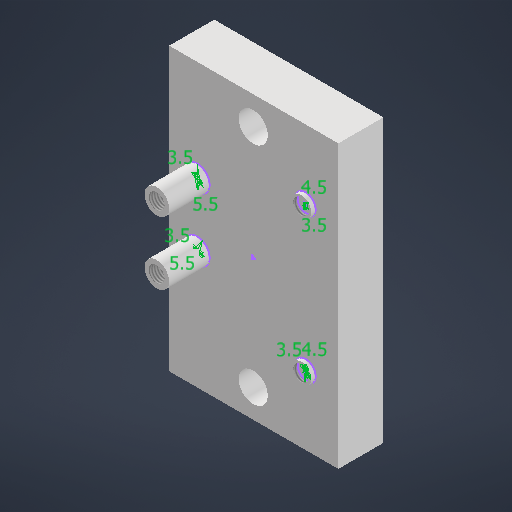
# Autodesk Inventor part: phm_top
Saved by Autodesk Inventor 2027 (Build 310192060, 192F)
## iProperties
Created: 2026-06-05
Part Number: phm_top
Material: Generic
Document SubType Name: Modeling
Designer: jacob
Density: 1 g/cm^3
Appearance: Default
Author: jacob
Autodesk Inventor part; units mm, degrees
ref_plane "YZ Plane" through (0, 0, 0) normal (1, 0, 0) x (0, 1, 0)
ref_plane "XZ Plane" through (0, 0, 0) normal (0, 1, 0) x (-1, 0, 0)
ref_plane "XY Plane" through (0, 0, 0) normal (0, 0, 1) x (1, 0, 0)
sketch "Sketch2" plane through (0, 0, 0) normal (0, 0, 1) x (1, 0, 0)
  line L0 (18.75, -31.25) -> (18.75, 31.25)
  line L1 (18.75, 31.25) -> (-18.75, 31.25)
  line L2 (-18.75, 31.25) -> (-18.75, -31.25)
  line L3 (-18.75, -31.25) -> (18.75, -31.25)
  circle A0 centre (-0.1179, 25) radius 3.25 projected
  circle A1 centre (-0.1179, -25) radius 3.25 projected
  point P0 (0, 0)
  constraints: 8 end point
extrude "Extrusion1" add sketch "Sketch2" along normal blind 10
sketch "Sketch4" plane through (0, 0, 10) normal (0, 0, 1) x (1, 0, 0)
  circle A0 centre (11.5, 16) radius 2.25
  circle A1 centre (-12.5, 9) radius 2.75
  circle A2 centre (-12.5, -5) radius 2.75
  circle A3 centre (11.5, -16) radius 2.25
  circle A4 centre (11.5, 16) radius 1.75
  circle A5 centre (11.5, -16) radius 1.75
  circle A6 centre (-12.5, -5) radius 1.75
  circle A7 centre (-12.5, 9) radius 1.75
  point P0 (0, 0)
  dimension "d6" = 3.5
  dimension "d7" = 3.5
  dimension "d8" = 3.5
  dimension "d9" = 3.5
  dimension "d10" = 4.5
  dimension "d11" = 4.5
  dimension "d12" = 5.5
  dimension "d13" = 5.5
  constraints: 8 centre point, 4 coincident
  measures "d6" diameter of A4
  measures "d7" diameter of A5
  measures "d8" diameter of A6
  measures "d9" diameter of A7
  measures "d10" diameter of A0
  measures "d11" diameter of A3
  measures "d12" diameter of A2
  measures "d13" diameter of A1
extrude "Extrusion2" add sketch "Sketch4" along normal blind 1 contours A0 | A3
extrude "Extrusion3" add sketch "Sketch4" along normal blind 9 contours A1 | A2
thread "Thread1" size "M3.5x0.6" class "6H" standard "ANSI Metric M Profile" full length
thread "Thread2" size "M3.5x0.6" class "6H" standard "ANSI Metric M Profile" full length
thread "Thread3" size "M3.5x0.6" class "6H" standard "ANSI Metric M Profile" full length
thread "Thread4" size "M3.5x0.6" class "6H" standard "ANSI Metric M Profile" full length
body "Solid1"
